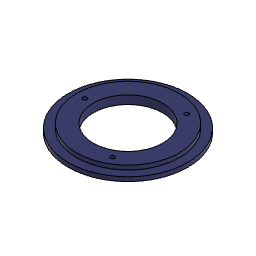
Cover+lock (Autodesk Fusion 360 design; units mm, degrees)
Autodesk Fusion 360 part; units mm, degrees
sketch "Sketch2" plane through (0, 0, 0) normal (0, 0, 1) x (1, 0, 0)
  line L0 (-61.4994, -0.2631) -> (-41.4992, -0.2631) construction
  circle A0 centre (-51.4994, -0.2631) radius 2.5
  circle A1 centre (0, 0) radius 41.5
  circle A2 centre (0, 0) radius 61.5
  circle A3 centre (0, 0) radius 71.5
  dimension "d13" = 83
  dimension "d14" = 20
  dimension "d36" = 5
  dimension "d49" = 10
  dimension "d17" = 10
  constraint coincident A1.centre A2.centre
  constraint concentric A1 A2
  constraint coincident L0.start A2
  constraint coincident L0.end A1
  constraint horizontal L0
  constraint coincident A0.centre L0
  constraint concentric A2 A3
  measures "d13" diameter of A1
  measures "d14" distance of A1 A2
  measures "d36" diameter of A0
  measures "d49" distance of A0.centre L0.start
  measures "d17" distance of A2 A3
extrude "Extrude3" add sketch "Sketch2" along normal blind 10 contours A2 makes body 1
extrude "Extrude4" add sketch "Sketch2" along normal blind 5 contours A3 bodies 1
pattern_circular "C-Pattern2" count 3 over 360 about axis through (0, 0, 1.75) along (0, 0, 1) of 1 faces at (-49.0025, -0.3877, 6.6667) on bodies 1
extrude "Extrude5" add sketch "Sketch2" against normal blind 5 separate body contours A2 | A3 makes body 2
move_body "Move1" bodies 2 to x (1, 0, 0) y (0, 1, 0) z (0, 0, 1) at (0, 0, 15)
pattern_circular "C-Pattern3" count 3 over 360 about axis through (0, 0, 1.75) along (0, 0, 1) of 1 faces at (-49.0025, -0.3877, 11.6667) on bodies 2
hidden bodies 2
